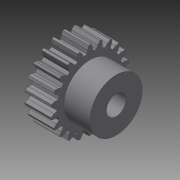
# Autodesk Inventor part: M-0.5 Zb-4mm M-0.7 Zb-5mm mN 21102200
Saved by Autodesk Inventor 2017.3 (Build 213256000, 256)
## iProperties
Category: PARTsolutions
Company: MAEDLER
Created: 2018-08-16
Part Number: M-0.5 Zb-4mm M-0.7 Zb-5mm mN 21102200
Material: Generic
Catalog Web Link: www.cadenas.de
Description: M-0.5 Zb-4mm M-0.7 Zb-5mm mN-Spur Gears, Steel, Module 0.5 and 0,7
Vendor: MAEDLER
Document SubType Name: Modeling
Designer: psadmin
Manufacturer: MAEDLER
Mass: 4 g
Surface Area: 6.08739 cm^2
Volume: 0.519365 cm^3
Density: 1 g/cm^3
Appearance: PSOLRGB-175-175-175
PSOL_IDENT_0: {$CADENAS_DATA\23d-libs\maedler\antriebselemente\stirnzahnraeder\stirnzahnraeder_stahl\modul_0.5_und
PSOL_IDENT_1: _0.7\m-0.5_zb-4mm_m-0.7_zb-5mm_mn.prj},237 {VTYP=3D},{NB=M-0.5 Zb-4mm M-0.7 Zb-5mm mN 21102200},{LIN
PSOL_IDENT_2: A=M-0.5 Zb-4mm M-0.7 Zb-5mm mN 21102200},{NN=M-0.5 Zb-4mm M-0.7 Zb-5mm mN},{DATE=27.10.2015 07:21:56
PSOL_IDENT_3: },{GEOMDATE=11.05.2009 09:51:00},{VERSION=},{LINEID=120},{WBVAR=},{WBNUMERIC=}  {NB=M-0.5 Zb-4mm M-0
PSOL_IDENT_4: .7 Zb-5mm mN 21102200},{LINA=M-0.5 Zb-4mm M-0.7 Zb-5mm mN 21102200},{KT=DUMMY},{ARTNR=21102200},{WST=
PSOL_IDENT_5: 11SMnPb30},{M=0.5},{Z=22},{PDF=PDF Katalogseite},{B1=4.0},{DA=12.00},{D=11.00},{NL=4},{ND=8},{B=3},{
PSOL_IDENT_6: MD=2.7},{GEW=4.000}
NN: M-0.5 Zb-4mm M-0.7 Zb-5mm mN
NT: Spur Gears, Steel, Module 0.5 and 0,7
NB: M-0.5 Zb-4mm M-0.7 Zb-5mm mN 21102200
NBSYN: M-0.5 Zb-4mm M-0.7 Zb-5mm mN $ARTNR.
LINA: M-0.5 Zb-4mm M-0.7 Zb-5mm mN 21102200
ARTNR: 21102200
WST: 11SMnPb30
M: 0.5
Z: 22
PDF: PDF Katalogseite
B1: 4
DA: 12
D: 11
NL: 4
ND: 8
B: 3
MD: 2.7
GEW: 4
SUPPLIER: MAEDLER
ARTICLENO: M-0.5 Zb-4mm M-0.7 Zb-5mm mN 21102200
BOMINFO: M-0.5 Zb-4mm M-0.7 Zb-5mm mN 21102200
CREATOR: CADENAS GmbH
Title: M-0.5 Zb-4mm M-0.7 Zb-5mm mN 21102200
Author: Cadenas PARTsolutions
Comments: Spur Gears, Steel, Module 0.5 and 0,7
Autodesk Inventor part; units mm, degrees
ref_plane "YZ Plane" through (0, 0, 0) normal (1, 0, 0) x (0, 1, 0)
ref_plane "XZ Plane" through (0, 0, 0) normal (0, 1, 0) x (-1, 0, 0)
ref_plane "XY Plane" through (0, 0, 0) normal (0, 0, 1) x (1, 0, 0)
sketch "Skizze_1" plane through (0, 0, 0) normal (1, 0, 0) x (0, 1, 0)
  arc A0 (0.1667, 5.9977) -> (-0.1667, 5.9977) centre (0, 0) ccw
  line L0 (-0.1667, 5.9977) -> (-0.3685, 5.4876)
  line L1 (-0.3685, 5.4876) -> (-0.4753, 4.9774)
  arc A1 (-0.4753, 4.9774) -> (-0.9463, 4.9096) centre (0, 0) ccw
  line L2 (-0.9463, 4.9096) -> (-1.1925, 5.3692)
  line L3 (-1.1925, 5.3692) -> (-1.5298, 5.8017)
  arc A2 (-1.5298, 5.8017) -> (-1.8497, 5.7078) centre (0, 0) ccw
  line L4 (-1.8497, 5.7078) -> (-1.8996, 5.1615)
  line L5 (-1.8996, 5.1615) -> (-1.8583, 4.6418)
  arc A3 (-1.8583, 4.6418) -> (-2.2911, 4.4442) centre (0, 0) ccw
  line L6 (-2.2911, 4.4442) -> (-2.6568, 4.8157)
  line L7 (-2.6568, 4.8157) -> (-3.1024, 5.1357)
  arc A4 (-3.1024, 5.1357) -> (-3.3828, 4.9555) centre (0, 0) ccw
  line L8 (-3.3828, 4.9555) -> (-3.2769, 4.4173)
  line L9 (-3.2769, 4.4173) -> (-3.0908, 3.9303)
  arc A5 (-3.0908, 3.9303) -> (-3.4504, 3.6187) centre (0, 0) ccw
  line L10 (-3.4504, 3.6187) -> (-3.906, 3.8721)
  line L11 (-3.906, 3.8721) -> (-4.4236, 4.0536)
  arc A6 (-4.4236, 4.0536) -> (-4.6419, 3.8017) centre (0, 0) ccw
  line L12 (-4.6419, 3.8017) -> (-4.3886, 3.3151)
  line L13 (-4.3886, 3.3151) -> (-4.0729, 2.9003)
  arc A7 (-4.0729, 2.9003) -> (-4.3301, 2.5) centre (0, 0) ccw
  line L14 (-4.3301, 2.5) -> (-4.8386, 2.6149)
  line L15 (-4.8386, 2.6149) -> (-5.3865, 2.6431)
  arc A8 (-5.3865, 2.6431) -> (-5.5249, 2.3399) centre (0, 0) ccw
  line L16 (-5.5249, 2.3399) -> (-5.1448, 1.9444)
  line L17 (-5.1448, 1.9444) -> (-4.725, 1.6353)
  arc A9 (-4.725, 1.6353) -> (-4.8591, 1.1788) centre (0, 0) ccw
  line L18 (-4.8591, 1.1788) -> (-5.3793, 1.1457)
  line L19 (-5.3793, 1.1457) -> (-5.9129, 1.0185)
  arc A10 (-5.9129, 1.0185) -> (-5.9604, 0.6886) centre (0, 0) ccw
  line L20 (-5.9604, 0.6886) -> (-5.4842, 0.4162)
  line L21 (-5.4842, 0.4162) -> (-4.9943, 0.2379)
  arc A11 (-4.9943, 0.2379) -> (-4.9943, -0.2379) centre (0, 0) ccw
  line L22 (-4.9943, -0.2379) -> (-5.4842, -0.4162)
  line L23 (-5.4842, -0.4162) -> (-5.9604, -0.6886)
  arc A12 (-5.9604, -0.6886) -> (-5.9129, -1.0185) centre (0, 0) ccw
  line L24 (-5.9129, -1.0185) -> (-5.3793, -1.1457)
  line L25 (-5.3793, -1.1457) -> (-4.8591, -1.1788)
  arc A13 (-4.8591, -1.1788) -> (-4.725, -1.6353) centre (0, 0) ccw
  line L26 (-4.725, -1.6353) -> (-5.1448, -1.9444)
  line L27 (-5.1448, -1.9444) -> (-5.5249, -2.3399)
  arc A14 (-5.5249, -2.3399) -> (-5.3865, -2.6431) centre (0, 0) ccw
  line L28 (-5.3865, -2.6431) -> (-4.8386, -2.6149)
  line L29 (-4.8386, -2.6149) -> (-4.3301, -2.5)
  arc A15 (-4.3301, -2.5) -> (-4.0729, -2.9003) centre (0, 0) ccw
  line L30 (-4.0729, -2.9003) -> (-4.3886, -3.3151)
  line L31 (-4.3886, -3.3151) -> (-4.6419, -3.8017)
  arc A16 (-4.6419, -3.8017) -> (-4.4236, -4.0536) centre (0, 0) ccw
  line L32 (-4.4236, -4.0536) -> (-3.906, -3.8721)
  line L33 (-3.906, -3.8721) -> (-3.4504, -3.6187)
  arc A17 (-3.4504, -3.6187) -> (-3.0908, -3.9303) centre (0, 0) ccw
  line L34 (-3.0908, -3.9303) -> (-3.2769, -4.4173)
  line L35 (-3.2769, -4.4173) -> (-3.3828, -4.9555)
  arc A18 (-3.3828, -4.9555) -> (-3.1024, -5.1357) centre (0, 0) ccw
  line L36 (-3.1024, -5.1357) -> (-2.6568, -4.8157)
  line L37 (-2.6568, -4.8157) -> (-2.2911, -4.4442)
  arc A19 (-2.2911, -4.4442) -> (-1.8583, -4.6418) centre (0, 0) ccw
  line L38 (-1.8583, -4.6418) -> (-1.8996, -5.1615)
  line L39 (-1.8996, -5.1615) -> (-1.8497, -5.7078)
  arc A20 (-1.8497, -5.7078) -> (-1.5298, -5.8017) centre (0, 0) ccw
  line L40 (-1.5298, -5.8017) -> (-1.1925, -5.3692)
  line L41 (-1.1925, -5.3692) -> (-0.9463, -4.9096)
  arc A21 (-0.9463, -4.9096) -> (-0.4753, -4.9774) centre (0, 0) ccw
  line L42 (-0.4753, -4.9774) -> (-0.3685, -5.4876)
  line L43 (-0.3685, -5.4876) -> (-0.1667, -5.9977)
  arc A22 (-0.1667, -5.9977) -> (0.1667, -5.9977) centre (0, 0) ccw
  line L44 (0.1667, -5.9977) -> (0.3685, -5.4876)
  line L45 (0.3685, -5.4876) -> (0.4753, -4.9774)
  arc A23 (0.4753, -4.9774) -> (0.9463, -4.9096) centre (0, 0) ccw
  line L46 (0.9463, -4.9096) -> (1.1925, -5.3692)
  line L47 (1.1925, -5.3692) -> (1.5298, -5.8017)
  arc A24 (1.5298, -5.8017) -> (1.8497, -5.7078) centre (0, 0) ccw
  line L48 (1.8497, -5.7078) -> (1.8996, -5.1615)
  line L49 (1.8996, -5.1615) -> (1.8583, -4.6418)
  arc A25 (1.8583, -4.6418) -> (2.2911, -4.4442) centre (0, 0) ccw
  line L50 (2.2911, -4.4442) -> (2.6568, -4.8157)
  line L51 (2.6568, -4.8157) -> (3.1024, -5.1357)
  arc A26 (3.1024, -5.1357) -> (3.3828, -4.9555) centre (0, 0) ccw
  line L52 (3.3828, -4.9555) -> (3.2769, -4.4173)
  line L53 (3.2769, -4.4173) -> (3.0908, -3.9303)
  arc A27 (3.0908, -3.9303) -> (3.4504, -3.6187) centre (0, 0) ccw
  line L54 (3.4504, -3.6187) -> (3.906, -3.8721)
  line L55 (3.906, -3.8721) -> (4.4236, -4.0536)
  arc A28 (4.4236, -4.0536) -> (4.6419, -3.8017) centre (0, 0) ccw
  line L56 (4.6419, -3.8017) -> (4.3886, -3.3151)
  line L57 (4.3886, -3.3151) -> (4.0729, -2.9003)
  arc A29 (4.0729, -2.9003) -> (4.3301, -2.5) centre (0, 0) ccw
  line L58 (4.3301, -2.5) -> (4.8386, -2.6149)
  line L59 (4.8386, -2.6149) -> (5.3865, -2.6431)
  arc A30 (5.3865, -2.6431) -> (5.5249, -2.3399) centre (0, 0) ccw
  line L60 (5.5249, -2.3399) -> (5.1448, -1.9444)
  line L61 (5.1448, -1.9444) -> (4.725, -1.6353)
  arc A31 (4.725, -1.6353) -> (4.8591, -1.1788) centre (0, 0) ccw
  line L62 (4.8591, -1.1788) -> (5.3793, -1.1457)
  line L63 (5.3793, -1.1457) -> (5.9129, -1.0185)
  arc A32 (5.9129, -1.0185) -> (5.9604, -0.6886) centre (0, 0) ccw
  line L64 (5.9604, -0.6886) -> (5.4842, -0.4162)
  line L65 (5.4842, -0.4162) -> (4.9943, -0.2379)
  arc A33 (4.9943, -0.2379) -> (4.9943, 0.2379) centre (0, 0) ccw
  line L66 (4.9943, 0.2379) -> (5.4842, 0.4162)
  line L67 (5.4842, 0.4162) -> (5.9604, 0.6886)
  arc A34 (5.9604, 0.6886) -> (5.9129, 1.0185) centre (0, 0) ccw
  line L68 (5.9129, 1.0185) -> (5.3793, 1.1457)
  line L69 (5.3793, 1.1457) -> (4.8591, 1.1788)
  arc A35 (4.8591, 1.1788) -> (4.725, 1.6353) centre (0, 0) ccw
  line L70 (4.725, 1.6353) -> (5.1448, 1.9444)
  line L71 (5.1448, 1.9444) -> (5.5249, 2.3399)
  arc A36 (5.5249, 2.3399) -> (5.3865, 2.6431) centre (0, 0) ccw
  line L72 (5.3865, 2.6431) -> (4.8386, 2.6149)
  line L73 (4.8386, 2.6149) -> (4.3301, 2.5)
  arc A37 (4.3301, 2.5) -> (4.0729, 2.9003) centre (0, 0) ccw
  line L74 (4.0729, 2.9003) -> (4.3886, 3.3151)
  line L75 (4.3886, 3.3151) -> (4.6419, 3.8017)
  arc A38 (4.6419, 3.8017) -> (4.4236, 4.0536) centre (0, 0) ccw
  line L76 (4.4236, 4.0536) -> (3.906, 3.8721)
  line L77 (3.906, 3.8721) -> (3.4504, 3.6187)
  arc A39 (3.4504, 3.6187) -> (3.0908, 3.9303) centre (0, 0) ccw
  line L78 (3.0908, 3.9303) -> (3.2769, 4.4173)
  line L79 (3.2769, 4.4173) -> (3.3828, 4.9555)
  arc A40 (3.3828, 4.9555) -> (3.1024, 5.1357) centre (0, 0) ccw
  line L80 (3.1024, 5.1357) -> (2.6568, 4.8157)
  line L81 (2.6568, 4.8157) -> (2.2911, 4.4442)
  arc A41 (2.2911, 4.4442) -> (1.8583, 4.6418) centre (0, 0) ccw
  line L82 (1.8583, 4.6418) -> (1.8996, 5.1615)
  line L83 (1.8996, 5.1615) -> (1.8497, 5.7078)
  arc A42 (1.8497, 5.7078) -> (1.5298, 5.8017) centre (0, 0) ccw
  line L84 (1.5298, 5.8017) -> (1.1925, 5.3692)
  line L85 (1.1925, 5.3692) -> (0.9463, 4.9096)
  arc A43 (0.9463, 4.9096) -> (0.4753, 4.9774) centre (0, 0) ccw
  line L86 (0.4753, 4.9774) -> (0.3685, 5.4876)
  line L87 (0.3685, 5.4876) -> (0.1667, 5.9977)
  constraints: 176 end point, 88 point on circle, 44 centre point
extrude "Extrusion1" add sketch "Skizze_1" along normal mid plane 4
sketch "Skizze_2" plane through (0, 0, 0) normal (0, 0, 1) x (1, 0, 0)
  line L0 (6, 0) -> (2, 0)
  line L1 (2, 0) -> (2, 4)
  line L2 (2, 4) -> (6, 4)
  line L3 (6, 4) -> (6, 0)
  line L4 (6, 0) -> (2, 0)
  constraints: 10 end point
revolve "Revolution1" add sketch "Skizze_2" angle 360 about axis through (6, 0, 0) along (1, 0, 0)
sketch "Skizze_3" plane through (6, 0, 0) normal (1, 0, 0) x (0, 1, 0)
  circle A0 centre (0, 0) radius 1.5
  constraints: 1 centre point
extrude "Extrusion2" cut sketch "Skizze_3" along normal mid plane 16
body "Solid1"
